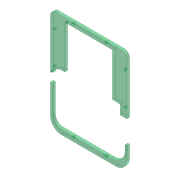
# Autodesk Inventor part: beagle_spacer_top
Saved by Autodesk Inventor 2014 (Build 180170000, 170)
## iProperties
Created: 2013-06-20
Part Number: beagle_spacer_top
Document SubType Name: Modeling
Designer: Administrator
Density: 1 g/cm^3
Mass: 9.21074 g
Surface Area: 80.6053 cm^2
Volume: 9.21074 cm^3
Material: Generic
Appearance: Clear - Green 1
Author: Administrator
Autodesk Inventor part; units mm, degrees
ref_plane "YZ Plane" through (0, 0, 0) normal (1, 0, 0) x (0, 1, 0)
ref_plane "XZ Plane" through (0, 0, 0) normal (0, 1, 0) x (-1, 0, 0)
ref_plane "XY Plane" through (0, 0, 0) normal (0, 0, 1) x (1, 0, 0)
sketch "Sketch1" plane through (0, 0, 0) normal (0, 0, 1) x (1, 0, 0)
  line L0 (9.8795, 48.1994) -> (9.8795, -53.4006)
  line L1 (16.2295, 54.5494) -> (92.4295, 54.5494)
  line L2 (98.7795, 48.1994) -> (98.7795, -53.4006)
  line L3 (22.5795, -66.1006) -> (86.0795, -66.1006)
  arc A0 (9.8795, -53.4006) -> (22.5795, -66.1006) centre (22.5795, -53.4006) ccw
  arc A1 (16.2295, 54.5494) -> (9.8795, 48.1994) centre (16.2295, 48.1994) ccw
  arc A2 (98.7795, 48.1994) -> (92.4295, 54.5494) centre (92.4295, 48.1994) ccw
  arc A3 (86.0795, -66.1006) -> (98.7795, -53.4006) centre (86.0795, -53.4006) ccw
  point P0 (0, 0)
  dimension "d0" = 12.7
  dimension "d1" = 6.35
  dimension "d2" = 120.65
  dimension "d3" = 88.9
  constraints: 8 end point, 8 point on circle, 8 tangent, 4 centre point, 2 equal radius, 1 horizontal, 1 vertical
  measures "d0" radius of A0
  measures "d1" radius of A1
  measures "d2" distance between parallel lines of L3 L1
  measures "d3" distance between parallel lines of L2 L0
extrude "Extrusion1" add sketch "Sketch1" along normal blind 3.175
sketch "Sketch2" plane through (0, 0, 3.175) normal (0, 0, 1) x (1, 0, 0)
  line L0 (9.8795, -53.4006) -> (9.8795, 48.1994) projected
  line L1 (98.7795, 48.1994) -> (98.7795, -53.4006) projected
  line L2 (16.2295, 54.5494) -> (92.4295, 54.5494) projected
  line L3 (26.6435, 49.4694) -> (82.0155, 49.4694)
  line L4 (82.0155, 49.4694) -> (82.0155, -1.3306)
  line L5 (82.0155, -1.3306) -> (26.6435, -1.3306)
  line L6 (26.6435, -1.3306) -> (26.6435, 49.4694)
  point P0 (0, 0)
  dimension "d13" = 16.764
  dimension "d14" = 16.764
  dimension "d15" = 5.08
  dimension "d16" = 55.88
  constraints: 8 end point
  measures "d13" distance between parallel lines of L0 L6
  measures "d14" distance between parallel lines of L1 L4
  measures "d15" distance between parallel lines of L2 L3
  measures "d16" distance between parallel lines of L5 L2
extrude "Extrusion2" cut sketch "Sketch2" against normal through all
sketch "Sketch8" plane through (0, 0, 3.175) normal (0, 0, 1) x (1, 0, 0)
  line L0 (82.0155, -1.3306) -> (26.6435, -1.3306) projected
  line L1 (9.8795, -53.4006) -> (9.8795, 48.1994) projected
  line L2 (98.7795, 48.1994) -> (98.7795, -53.4006) projected
  line L3 (18.7695, -2.6006) -> (86.0795, -2.6006)
  line L4 (12.3173, -6.9948) -> (9.8795, -6.9948)
  arc A0 (86.1117, -10.6693) -> (86.0795, -10.656) centre (83.9402, -15.8848) ccw
  line L5 (86.0795, -66.1006) -> (22.5795, -66.1006) projected
  arc A1 (18.7695, -2.6006) -> (12.3173, -6.9948) centre (18.7695, -9.5348) ccw
  arc A2 (9.8795, -51.4448) -> (18.7695, -60.3348) centre (18.7695, -51.4448) ccw
  arc A3 (86.0795, -60.3348) -> (98.7795, -53.519) centre (86.0795, -45.0948) ccw
  line L6 (86.0795, -60.3348) -> (18.7695, -60.3348)
  arc A4 (98.7795, -15.3006) -> (86.0795, -2.6006) centre (86.0795, -15.3006) ccw
  line L7 (9.8795, -6.9948) -> (9.8795, -51.4448)
  line L8 (98.7795, -15.3006) -> (98.7795, -53.519)
  point P0 (0, 0)
  dimension "d70" = 1.27
  dimension "d89" = 8.89
  dimension "d90" = 56.5658
  dimension "d95" = 8.89
  dimension "d96" = 14.6558
  dimension "d101" = 12.7
  dimension "d102" = 21.0058
  dimension "d103" = 12.7
  dimension "d104" = 50.2158
  dimension "d105" = 5.7658
  dimension "d107" = 59.1058
  constraints: 10 end point, 10 point on circle, 5 centre point, 5 tangent, 4 point on line, 2 horizontal
  measures "d70" distance between parallel lines of L0 L3
  measures "d89" distance from line of L1 A1.centre
  measures "d90" distance from line of L5 A1.centre
  measures "d95" distance from line of L1 A2.centre
  measures "d96" distance from line of L5 A2.centre
  measures "d101" distance from line of L2 A3.centre
  measures "d102" distance from line of L5 A3.centre
  measures "d103" distance from line of L2 A4.centre
  measures "d104" distance from line of L5 A0.centre
  measures "d105" distance between parallel lines of L5 L6
  measures "d107" distance between parallel lines of L5 L4
extrude "Extrusion16" [suppressed]
sketch "Sketch9" plane through (0, 0, 3.175) normal (0, 0, 1) x (1, 0, 0)
  line L0 (9.8795, -53.4006) -> (9.8795, 48.1994) projected
  line L1 (86.0795, -66.1006) -> (22.5795, -66.1006) projected
  line L2 (98.7795, 48.1994) -> (98.7795, -53.4006) projected
  arc A0 (18.7695, -3.1848) -> (12.4195, -9.5348) centre (18.7695, -9.5348) ccw
  arc A1 (98.7795, -15.8848) -> (98.1266, -11.8651) centre (86.0795, -15.8848) ccw
  arc A2 (12.4195, -51.4448) -> (18.7695, -57.7948) centre (18.7695, -51.4448) ccw
  arc A3 (86.0795, -57.7948) -> (91.1595, -56.7345) centre (86.0795, -45.0948) ccw
  line L3 (18.7695, -3.1848) -> (86.0795, -3.1848)
  line L4 (98.7795, -15.8848) -> (98.7795, -38.9988)
  line L5 (86.0795, -57.7948) -> (18.7695, -57.7948)
  line L6 (12.4195, -51.4448) -> (12.4195, -9.5348)
  arc A4 (101.3195, -15.8848) -> (100.7798, -11.8651) centre (86.0795, -15.8848) ccw
  line L7 (101.3195, -15.8848) -> (101.3195, -38.9988)
  arc A5 (86.0795, -60.3348) -> (98.7795, -53.519) centre (86.0795, -45.0948) ccw
  line L8 (86.0795, -60.3348) -> (81.5075, -60.3348)
  arc A6 (9.8795, -51.4448) -> (18.7695, -60.3348) centre (18.7695, -51.4448) ccw
  line L9 (9.8795, -51.4448) -> (9.8795, -9.5348)
  arc A7 (18.7695, -0.6448) -> (9.9707, -8.2648) centre (18.7695, -9.5348) ccw
  line L10 (18.7695, -0.6448) -> (86.0795, -0.6448)
  line L11 (9.8795, -8.2648) -> (12.4195, -8.2648)
  arc A8 (12.4195, -51.4448) -> (21.3095, -60.3348) centre (21.3095, -51.4448) ccw
  line L12 (9.8795, -19.0598) -> (12.4195, -19.0598)
  arc A9 (23.0444, -0.6448) -> (13.1925, -6.4985) centre (23.0444, -11.8621) ccw
  line L13 (91.1595, -11.8651) -> (96.7475, -11.8651)
  line L14 (91.1595, -11.8651) -> (91.1595, -4.2451)
  line L15 (91.1595, -4.2451) -> (91.1595, -1.5164)
  line L16 (98.7795, -11.8651) -> (100.7798, -11.8651)
  line L17 (96.7475, -38.9988) -> (96.7475, -45.0948)
  line L18 (96.7475, -38.9988) -> (98.7795, -38.9988)
  arc A10 (81.5075, -60.3348) -> (89.9317, -57.7948) centre (81.5075, -45.0948) ccw
  arc A11 (91.5546, -56.554) -> (96.7475, -45.0948) centre (81.5075, -45.0948) ccw
  arc A12 (91.5546, -56.554) -> (96.7475, -51.9857) centre (86.0795, -45.0948) ccw
  arc A13 (13.1925, -6.4985) -> (12.4195, -8.2648) centre (23.0444, -11.8621) ccw
  arc A14 (9.9707, -8.2648) -> (9.8795, -9.5348) centre (18.7695, -9.5348) ccw
  arc A15 (91.1595, -1.5164) -> (86.0795, -0.6448) centre (86.0795, -15.8848) ccw
  arc A16 (98.1266, -11.8651) -> (91.1595, -4.2451) centre (86.0795, -15.8848) ccw
  arc A17 (91.1595, -56.7345) -> (91.5546, -56.554) centre (86.0795, -45.0948) ccw
  arc A18 (96.7475, -51.9857) -> (98.7795, -45.0948) centre (86.0795, -45.0948) ccw
  arc A19 (89.9317, -57.7948) -> (91.5546, -56.554) centre (81.5075, -45.0948) ccw
  line L19 (81.5075, -60.3348) -> (18.7695, -60.3348)
  line L20 (98.1266, -11.8651) -> (98.7795, -11.8651)
  arc A20 (98.7795, -7.4606) -> (91.1595, -1.5164) centre (86.0795, -15.8848) ccw
  arc A21 (91.1595, -4.2451) -> (86.0795, -3.1848) centre (86.0795, -15.8848) ccw
  arc A22 (98.7795, -53.519) -> (101.3195, -45.0948) centre (86.0795, -45.0948) ccw
  line L21 (101.3195, -38.9988) -> (101.3195, -45.0948)
  arc A23 (100.7798, -11.8651) -> (98.7795, -7.4606) centre (86.0795, -15.8848) ccw
  line L22 (96.7475, -11.8651) -> (98.1266, -11.8651)
  line L23 (98.7795, -38.9988) -> (98.7795, -45.0948)
  line L24 (98.7795, -11.8651) -> (98.7795, -15.8848)
  point P0 (0, 0)
  dimension "d110" = 6.35
  dimension "d111" = 6.35
  dimension "d112" = 12.7
  dimension "d113" = 12.7
  dimension "d114" = 54.61
  dimension "d115" = 86.36
  dimension "d116" = 8.3058
  dimension "d122" = 10.795
  dimension "d123" = 5.08
  dimension "d127" = 7.62
  dimension "d128" = 7.62
  dimension "d129" = 2.032
  dimension "d130" = 18.796
  constraints: 52 point on circle, 44 end point, 34 tangent, 24 centre point, 16 point on line, 7 horizontal, 5 vertical, 3 collinear, 1 horizontal alignment, 1 other
  measures "d110" radius of A0
  measures "d111" radius of A2
  measures "d112" radius of A3
  measures "d113" radius of A1
  measures "d114" distance between parallel lines of L5 L3
  measures "d115" distance between parallel lines of L4 L6
  measures "d116" distance between parallel lines of L1 L5
  measures "d122" distance between parallel lines of L11 L12
  measures "d123" distance between parallel lines of L3 L11
  measures "d127" distance of L13.start L16.start
  measures "d128" distance of L13.start L14.end
  measures "d129" distance between parallel lines of L2 L17
  measures "d130" distance from line of L5 L17.start
extrude "Extrusion21" cut sketch "Sketch9" against normal through all contours L0 A14 L11 A13 A0 L6 L12 | L6 A0 L3 A21 L14 L13 L22 A1 L2 L18 L17 A11 A17 A3 L5 A2 | A8 A2 L5 A3 A17 A19 A10 L19 | A9 L10 A15 L15 A21 L3 A0 | L20 L2 A1
sketch "Sketch11" plane through (0, 0, 3.175) normal (0, 0, 1) x (1, 0, 0)
  line L0 (98.7795, 48.1994) -> (98.7795, -11.8651) projected
  line L1 (16.2295, 54.5494) -> (92.4295, 54.5494) projected
  line L2 (9.8795, -9.5348) -> (9.8795, 48.1994) projected
  circle A0 centre (13.0037, 35.4994) radius 1.27
  circle A1 centre (13.0037, -2.6006) radius 1.27
  circle A2 centre (35.2795, 51.4252) radius 1.27
  circle A3 centre (73.3795, 51.4252) radius 1.27
  circle A4 centre (95.6553, 35.4994) radius 1.27
  circle A5 centre (95.6553, -2.6006) radius 1.27
  circle A6 centre (35.2795, -62.9764) radius 1.27
  circle A7 centre (73.3795, -62.9764) radius 1.27
  line L3 (86.0795, -66.1006) -> (22.5795, -66.1006) projected
  point P0 (0, 0)
  dimension "d135" = 3.1242
  dimension "d136" = 3.1242
  dimension "d137" = 3.1242
  dimension "d138" = 3.1242
  dimension "d139" = 2.54
  dimension "d140" = 25.4
  dimension "d141" = 19.05
  dimension "d142" = 38.1
  dimension "d143" = 38.1
  constraints: 8 centre point, 7 equal radius, 4 horizontal alignment, 4 vertical alignment
  measures "d135" distance from line of L2 A0.centre
  measures "d136" distance from line of L0 A4.centre
  measures "d137" distance from line of L1 A2.centre
  measures "d138" distance from line of L3 A6.centre
  measures "d139" diameter of A2
  measures "d140" distance from line of L2 A2.centre
  measures "d141" distance from line of L1 A0.centre
  measures "d142" distance of A3.centre A2.centre
  measures "d143" distance of A1.centre A0.centre
extrude "Extrusion22" cut sketch "Sketch11" against normal through all
equation "\"d14\" = d13"
body "Solid1"
